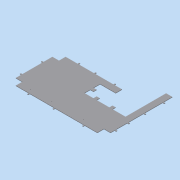
# Autodesk Inventor part: tx_v2_04_cu_shield_no-folds
Saved by Autodesk Inventor 2014 (Build 180170000, 170)
## iProperties
Created: 2014-03-05
Part Number: tx_v2_04_cu_shield_no-folds
Material: Generic
Document SubType Name: Sheet Metal
Designer: Robert Davis
Density: 1 g/cm^3
Sheet Metal Rule: Default_mm
Appearance: Default
Flat Pattern Width: 6.62019 cm
Flat Pattern Length: 9.2582 cm
Flat Pattern Area: 61.291 cm^2
Sheet Metal Width: 66.2019 mm
Sheet Metal Length: 92.5820 mm
Sheet Metal Area: 6129.1043 mm^2
Author: Robert Davis
Autodesk Inventor part; units mm, degrees
ref_plane "YZ Plane" through (0, 0, 0) normal (1, 0, 0) x (0, 1, 0)
ref_plane "XZ Plane" through (0, 0, 0) normal (0, 1, 0) x (-1, 0, 0)
ref_plane "XY Plane" through (0, 0, 0) normal (0, 0, 1) x (1, 0, 0)
sketch "Sketch1" plane through (0, 0, 0) normal (0, 0, 1) x (1, 0, 0)
  line L0 (7.5, 46.3001) -> (22.25, 46.3001)
  line L1 (22.25, 46.3001) -> (22.25, 52.2431)
  line L2 (-31.08, 52.2431) -> (-31.08, 45.9911)
  line L3 (-31.08, 45.9911) -> (-37.332, 45.9911)
  line L4 (-37.332, 11.4131) -> (-31.08, 11.4131)
  line L5 (-31.08, 11.4131) -> (-31.08, 5.1611)
  line L6 (45.998, 5.1611) -> (45.998, 11.4131)
  line L7 (45.998, 11.4131) -> (52.25, 11.4131)
  line L8 (52.25, 69.863) -> (46.307, 69.863)
  line L9 (46.307, 69.863) -> (46.307, 31.493)
  line L10 (-17.791, 5.1611) -> (-17.791, 3.6611)
  line L11 (-17.791, 3.6611) -> (-18.791, 3.6611)
  line L12 (-18.791, 3.6611) -> (-18.791, 5.1611)
  line L13 (6.209, 5.1611) -> (6.209, 3.6611)
  line L14 (6.209, 3.6611) -> (5.209, 3.6611)
  line L15 (5.209, 3.6611) -> (5.209, 5.1611)
  line L16 (34.209, 5.1611) -> (34.209, 3.6611)
  line L17 (34.209, 3.6611) -> (33.209, 3.6611)
  line L18 (33.209, 3.6611) -> (33.209, 5.1611)
  line L19 (-31.08, 5.1611) -> (-18.791, 5.1611)
  line L20 (34.209, 5.1611) -> (45.998, 5.1611)
  line L21 (-17.791, 5.1611) -> (5.209, 5.1611)
  line L22 (6.209, 5.1611) -> (33.209, 5.1611)
  line L23 (-37.332, 16.7021) -> (-38.832, 16.7021)
  line L24 (-38.832, 16.7021) -> (-38.832, 17.7021)
  line L25 (-38.832, 17.7021) -> (-37.332, 17.7021)
  line L26 (-37.332, 36.7021) -> (-38.832, 36.7021)
  line L27 (-38.832, 36.7021) -> (-38.832, 37.7021)
  line L28 (-38.832, 37.7021) -> (-37.332, 37.7021)
  line L29 (-18.791, 52.2431) -> (-18.791, 53.7431)
  line L30 (-18.791, 53.7431) -> (-19.791, 53.7431)
  line L31 (-19.791, 53.7431) -> (-19.791, 52.2431)
  line L32 (-3.291, 52.2431) -> (-3.291, 53.7431)
  line L33 (-3.291, 53.7431) -> (-4.291, 53.7431)
  line L34 (-4.291, 53.7431) -> (-4.291, 52.2431)
  line L35 (-4.291, 52.2431) -> (-18.791, 52.2431)
  line L36 (-19.791, 52.2431) -> (-31.08, 52.2431)
  line L37 (-37.332, 45.9911) -> (-37.332, 37.7021)
  line L38 (-37.332, 36.7021) -> (-37.332, 17.7021)
  line L39 (-37.332, 16.7021) -> (-37.332, 11.4131)
  line L40 (15.091, 52.2431) -> (15.091, 53.7431)
  line L41 (15.091, 53.7431) -> (14.091, 53.7431)
  line L42 (14.091, 53.7431) -> (14.091, 52.2431)
  line L43 (52.25, 15.2021) -> (53.75, 15.2021)
  line L44 (53.75, 15.2021) -> (53.75, 16.2021)
  line L45 (53.75, 16.2021) -> (52.25, 16.2021)
  line L46 (52.25, 27.2021) -> (53.75, 27.2021)
  line L47 (53.75, 27.2021) -> (53.75, 28.2021)
  line L48 (53.75, 28.2021) -> (52.25, 28.2021)
  line L49 (52.25, 42.5821) -> (53.75, 42.5821)
  line L50 (53.75, 42.5821) -> (53.75, 43.5821)
  line L51 (53.75, 43.5821) -> (52.25, 43.5821)
  line L52 (52.25, 60.5821) -> (53.75, 60.5821)
  line L53 (53.75, 60.5821) -> (53.75, 61.5821)
  line L54 (53.75, 61.5821) -> (52.25, 61.5821)
  line L55 (22.25, 52.2431) -> (15.091, 52.2431)
  line L56 (14.091, 52.2431) -> (-3.291, 52.2431)
  line L57 (52.25, 61.5821) -> (52.25, 69.863)
  line L58 (52.25, 43.5821) -> (52.25, 60.5821)
  line L59 (52.25, 11.4131) -> (52.25, 15.2021)
  line L60 (52.25, 16.2021) -> (52.25, 27.2021)
  line L61 (52.25, 28.2021) -> (52.25, 42.5821)
  line L62 (7.5, 39.993) -> (10.5, 39.993)
  line L63 (10.5, 39.993) -> (10.5, 36.993)
  line L64 (10.5, 36.993) -> (7.5, 36.993)
  line L65 (31, 31.493) -> (31, 34.493)
  line L66 (31, 34.493) -> (34, 34.493)
  line L67 (34, 34.493) -> (34, 31.493)
  line L68 (16, 31.493) -> (16, 34.493)
  line L69 (16, 34.493) -> (19, 34.493)
  line L70 (19, 34.493) -> (19, 31.493)
  line L71 (7.5, 31.493) -> (7.5, 36.993)
  line L72 (7.5, 39.993) -> (7.5, 46.3001)
  line L73 (34, 31.493) -> (46.307, 31.493)
  line L74 (7.5, 31.493) -> (16, 31.493)
  line L75 (19, 31.493) -> (31, 31.493)
  circle A0 centre (-21.08, 9.1611) radius 0.25
  circle A1 centre (-1.08, 9.1611) radius 0.25
  circle A2 centre (28.92, 9.1611) radius 0.25
  point P0 (0, 0)
  point P1 (-18.291, 3.6611)
  point P2 (5.709, 3.6611)
  point P3 (33.709, 3.6611)
  point P4 (-38.832, 17.2021)
  point P5 (-38.832, 37.2021)
  point P6 (-19.291, 53.7431)
  point P7 (-3.791, 53.7431)
  point P8 (14.591, 53.7431)
  point P9 (53.75, 61.0821)
  point P10 (53.75, 43.0821)
  point P11 (53.75, 27.7021)
  point P12 (53.75, 15.7021)
  point P13 (10.5, 38.493)
  point P14 (17.5, 34.493)
  point P15 (32.5, 34.493)
  dimension "d3" = 14.75
  dimension "d4" = 14.8071
  dimension "d5" = 6.252
  dimension "d7" = 34.578
  dimension "d8" = 77.078
  dimension "d9" = 38.37
  dimension "d10" = 5.943
  dimension "d60" = 5.943
  dimension "d74" = 1.5
  dimension "d75" = 1
  dimension "d76" = 12.789
  dimension "d77" = 24
  dimension "d78" = 28
  dimension "d79" = 5.789
  dimension "d80" = 20
  dimension "d81" = 11.789
  dimension "d82" = 15.5
  dimension "d83" = 4.289
  dimension "d84" = 12
  dimension "d85" = 15.38
  dimension "d86" = 18
  dimension "d87" = 18.382
  dimension "d89" = 38.58
  dimension "d90" = 7.5
  dimension "d91" = 31.493
  dimension "d92" = 3
  dimension "d93" = 3
  dimension "d94" = 7
  dimension "d95" = 10
  dimension "d96" = 15
  dimension "d117" = 0.5
  dimension "d118" = 20
  dimension "d119" = 30
  dimension "d120" = 10
  dimension "d121" = 4
  constraints: 152 end point, 46 equal length, 31 horizontal, 23 vertical, 15 midpoint, 15 parallel, 7 perpendicular, 3 centre point, 2 equal radius
  measures "d3" distance of L0.start L0.end
  measures "d4" distance of L71.start L0.start
  measures "d5" distance of L2.start L2.end
  measures "d7" distance of L3.end L4.start
  measures "d8" distance of L5.end L6.start
  measures "d9" distance of L8.end L9.end
  measures "d10" distance of L0.end L1.end
  measures "d60" distance of L8.start L8.end
  measures "d74" distance of L11.end L12.end
  measures "d75" distance of L10.end L11.end
  measures "d76" distance from line of point (-18.291, 3.661) L5
  measures "d77" distance of point (5.709, 3.661) point (-18.291, 3.661)
  measures "d78" distance of point (33.709, 3.661) point (5.709, 3.661)
  measures "d79" distance from line of point (-38.832, 17.202) L4
  measures "d80" distance of point (-38.832, 37.202) point (-38.832, 17.202)
  measures "d81" distance from line of point (-19.291, 53.743) L2
  measures "d82" distance of point (-3.791, 53.743) point (-19.291, 53.743)
  measures "d83" distance from line of point (53.75, 15.702) L7
  measures "d84" distance of point (53.75, 27.702) point (53.75, 15.702)
  measures "d85" distance of point (53.75, 43.082) point (53.75, 27.702)
  measures "d86" distance of point (53.75, 61.082) point (53.75, 43.082)
  measures "d87" distance of point (14.591, 53.743) point (-3.791, 53.743)
  measures "d89" distance between parallel lines of L2 L72
  measures "d90" distance from line of point (0, 0) L71
  measures "d91" distance from line of point (0, 0) L74
  measures "d92" distance of L62.end L63.end
  measures "d93" distance of L62.start L62.end
  measures "d94" distance from line of point (10.5, 38.493) L74
  measures "d95" distance from line of point (17.5, 34.493) L71
  measures "d96" distance of point (32.5, 34.493) point (17.5, 34.493)
  measures "d117" diameter of A0
  measures "d118" distance of A1.centre A0.centre
  measures "d119" distance of A2.centre A1.centre
  measures "d120" distance from line of A0.centre L5
  measures "d121" distance from line of A0.centre L19
extrude "Plate1" add sketch "Sketch1" along normal blind 0.381
sketch "Sketch4" plane through (0, 0, 0) normal (0, 0, -1) x (-1, 0, 0)
  line L0 (-7.5, 31.493) -> (-7.5, 46.3001) projected
  line L1 (31.08, 52.2431) -> (31.08, 45.9911) projected
  line L2 (31.08, 46.1431) -> (-7.5, 46.1431)
  line L3 (-22.25, 52.2431) -> (31.08, 52.2431) projected
  point P0 (0, 0)
  dimension "d61" = 6.1
  constraints: 2 end point, 2 point on line, 1 horizontal
  measures "d61" distance between parallel lines of L3 L2
feature "Fold2" [suppressed]
sketch "Sketch5" plane through (-31.08, 52.2431, 0) normal (0, 0, -1) x (1, 0, 0)
  line L0 (53.33, 0) -> (0, 0) projected
  line L1 (38.58, 5.943) -> (53.33, 5.943) projected
  line L2 (38.73, 5.943) -> (38.73, 0)
  line L3 (53.33, 5.943) -> (53.33, 0) projected
  point P0 (31.08, 52.2431)
  dimension "d62" = 14.6
  constraints: 2 end point, 2 point on line, 1 vertical
  measures "d62" distance between parallel lines of L2 L3
feature "Fold3" [suppressed]
sketch "Sketch6" plane through (0, 0, 0) normal (0, 0, -1) x (-1, 0, 0)
  line L0 (37.332, 11.4131) -> (31.08, 11.4131) projected
  line L1 (31.08, 45.9911) -> (37.332, 45.9911) projected
  line L2 (31.232, 45.9911) -> (31.232, 11.4131)
  line L3 (37.332, 45.9911) -> (37.332, 11.4131) projected
  point P0 (0, 0)
  dimension "d63" = 6.1
  constraints: 2 end point, 2 point on line, 1 vertical
  measures "d63" distance between parallel lines of L3 L2
feature "Fold4" [suppressed]
sketch "Sketch7" plane through (0, 0, 0) normal (0, 0, -1) x (-1, 0, 0)
  line L0 (-45.998, 5.1611) -> (-45.998, 11.4131) projected
  line L1 (31.08, 11.4131) -> (31.08, 5.1611) projected
  line L2 (-45.998, 11.2611) -> (31.08, 11.2611)
  line L3 (31.08, 5.1611) -> (-45.998, 5.1611) projected
  point P0 (0, 0)
  dimension "d64" = 6.1
  constraints: 2 end point, 2 point on line, 1 horizontal
  measures "d64" distance between parallel lines of L3 L2
feature "Fold5" [suppressed]
sketch "Sketch8" plane through (0, 0, 0) normal (0, 0, -1) x (-1, 0, 0)
  line L0 (-46.307, 31.493) -> (-7.5, 31.493) projected
  line L1 (-45.998, 11.4131) -> (-52.25, 11.4131) projected
  line L2 (-46.15, 11.4131) -> (-46.15, 31.493)
  line L3 (-52.25, 11.4131) -> (-52.25, 69.863) projected
  point P0 (0, 0)
  dimension "d65" = 6.1
  constraints: 2 end point, 2 point on line, 1 vertical
  measures "d65" distance between parallel lines of L2 L3
feature "Fold6" [suppressed]
sketch "Sketch9" plane through (52.25, 11.4131, 0) normal (0, 0, -1) x (-1, 0, 0)
  line L0 (5.943, 58.4499) -> (5.943, 20.0799) projected
  line L1 (0, 0) -> (0, 58.4499) projected
  line L2 (5.943, 20.2299) -> (0, 20.2299)
  line L3 (0, 58.4499) -> (5.943, 58.4499) projected
  point P0 (52.25, -11.4131)
  dimension "d66" = 38.22
  constraints: 2 end point, 2 point on line, 1 horizontal
  measures "d66" distance between parallel lines of L3 L2
feature "Fold7" [suppressed]
ref_plane "Work Plane1" through (-31.08, 5.1611, 0.1905) normal (0, 0, -1) x (1, 0, 0)
ref_plane "Work Plane2" through (-37.332, 11.4131, 0.1905) normal (0, 0, -1) x (-1, 0, 0)
ref_plane "Work Plane3" through (-31.08, 52.2431, 0.1905) normal (0, 0, 1) x (1, 0, 0)
ref_plane "Work Plane4" through (52.25, 11.4131, 0.1905) normal (0, 0, 1) x (1, 0, 0)
ref_plane "Work Plane5" through (22.25, 52.2431, 0.1905) normal (0, 0, 1) x (0, 1, 0)
ref_plane "Work Plane6" through (52.25, 69.863, 0.1905) normal (0, 0, -1) x (0, -1, 0)
ref_plane "Work Plane7" through (-18.291, 3.6611, 0.381) normal (-1, 0, 0) x (0, 1, 0)
ref_plane "Work Plane8" through (5.709, 3.6611, 0.381) normal (-1, 0, 0) x (0, 1, 0)
ref_plane "Work Plane9" through (33.709, 3.6611, 0.381) normal (-1, 0, 0) x (0, 1, 0)
ref_plane "Work Plane10" through (53.75, 15.7021, 0.381) normal (0, -1, 0) x (0, 0, 1)
ref_plane "Work Plane11" through (53.75, 27.7021, 0.381) normal (0, -1, 0) x (0, 0, 1)
ref_plane "Work Plane12" through (53.75, 43.0821, 0.381) normal (0, -1, 0) x (1, 0, 0)
ref_plane "Work Plane13" through (53.75, 61.0821, 0.381) normal (0, -1, 0) x (1, 0, 0)
ref_plane "Work Plane14" through (14.591, 53.7431, 0.381) normal (-1, 0, 0) x (0, 0, 1)
ref_plane "Work Plane15" through (-3.791, 53.7431, 0.381) normal (-1, 0, 0) x (0, -1, 0)
ref_plane "Work Plane16" through (-19.291, 53.7431, 0.381) normal (-1, 0, 0) x (0, -1, 0)
ref_plane "Work Plane17" through (-38.832, 37.2021, 0.381) normal (0, 1, 0) x (0, 0, -1)
ref_plane "Work Plane18" through (-38.832, 17.2021, 0.381) normal (0, 1, 0) x (0, 0, -1)
sketch "Sketch11" plane through (0, 0, 0) normal (0, 0, -1) x (-1, 0, 0)
  line L0 (-10.5, 39.993) -> (-7.5, 39.993) projected
  line L1 (-10.5, 36.993) -> (-10.5, 39.993) projected
  line L2 (-7.5, 36.993) -> (-10.5, 36.993) projected
  line L3 (-8.032, 36.993) -> (-8.032, 39.993)
  point P0 (0, 0)
  dimension "d97" = 2.468
  constraints: 2 end point, 2 point on line, 1 vertical
  measures "d97" distance between parallel lines of L3 L1
feature "Fold8" [suppressed]
sketch "Sketch12" plane through (0, 0, 0) normal (0, 0, -1) x (-1, 0, 0)
  line L0 (-16, 34.493) -> (-16, 31.493) projected
  line L1 (-34, 34.493) -> (-31, 34.493) projected
  line L2 (-34, 31.493) -> (-34, 34.493) projected
  line L3 (-16, 32.025) -> (-34, 32.025)
  point P0 (0, 0)
  dimension "d104" = 2.468
  constraints: 2 end point, 2 point on line, 1 horizontal
  measures "d104" distance between parallel lines of L3 L1
feature "Fold10" [suppressed]
equation "\"d19\" = BendReliefWidth"
equation "\"d20\" = BendReliefDepth"
equation "\"d21\" = MinimumRemnant"
equation "\"d22\" = BendRadius"
equation "\"d24\" = BendRadius"
equation "\"d26\" = BendReliefWidth"
equation "\"d27\" = BendReliefDepth"
equation "\"d28\" = MinimumRemnant"
equation "\"d29\" = BendRadius"
equation "\"d31\" = BendRadius"
equation "\"d33\" = BendReliefWidth"
equation "\"d34\" = BendReliefDepth"
equation "\"d35\" = MinimumRemnant"
equation "\"d36\" = BendRadius"
equation "\"d38\" = BendRadius"
equation "\"d40\" = BendReliefWidth"
equation "\"d41\" = BendReliefDepth"
equation "\"d42\" = MinimumRemnant"
equation "\"d43\" = BendRadius"
equation "\"d45\" = BendRadius"
equation "\"d47\" = BendReliefWidth"
equation "\"d48\" = BendReliefDepth"
equation "\"d49\" = MinimumRemnant"
equation "\"d50\" = BendRadius"
equation "\"d52\" = BendRadius"
equation "\"d54\" = BendReliefWidth"
equation "\"d55\" = BendReliefDepth"
equation "\"d56\" = MinimumRemnant"
equation "\"d57\" = BendRadius"
equation "\"d59\" = BendRadius"
equation "\"BendReliefWidth\" = Thickness"
equation "\"BendReliefDepth\" = 0.5 * Thickness"
equation "\"CornerReliefSize\" = 4 * Thickness"
equation "\"MinimumRemnant\" = 2 * Thickness"
equation "\"TransitionRadius\" = BendRadius"
equation "\"JacobiRadiusSize\" = BendRadius"
equation "\"GapSize\" = Thickness"
equation "\"d11\" = BendRadius"
equation "\"BendRadius\" = 0.001"
equation "\"Thickness\" = 0.381"
body "Solid1"
